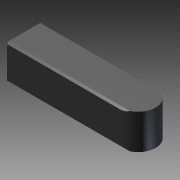
# Autodesk Inventor part: KEGS4-15
Saved by Autodesk Inventor 2011 SP1 (Build 150282100, 282)
## iProperties
Created: 2016-04-02
Part Number: KEGS4-15
Catalog Web Link: www.cadenas.de
Description: KED, KEDH, KEDS, KES, KESH, KESS, KEG, KEGH, KEGS-Parallel Keys
Vendor: MISUMI
Document SubType Name: Modeling
Designer: psAdmin
Manufacturer: MISUMI
Mass: 0.232054 g
Surface Area: 2.55242 cm^2
Volume: 0.232054 cm^3
Density: 1 g/cm^3
Category: PARTsolutions
Company: MISUMI
Title: KEGS4-15
Author: Cadenas PARTsolutions
Comments: Parallel Keys
PSOL_IDENT_0: {$CADENAS_DATA\23d-libs\misumi\metric\28_keys_magnets\kegh.prj},214 {VTYP=3D},{NB=KEGS4-15},{LINA=KE
PSOL_IDENT_1: GS4-15},{NN=KED, KEDH, KEDS, KES, KESH, KESS, KEG, KEGH, KEGS},{DATE=03.06.2015 11:36:45},{GEOMDATE=
PSOL_IDENT_2: 22.08.2013},{VERSION=},{LINEID=30},{LINESUBID=-1},{WBVAR=TYS,MAT,HARD,L,ALT1,LC}  {NB=KEGS4-15},{LIN
PSOL_IDENT_3: A=KEGS4-15},{KT=DUMMY},{PN=KEGS4-15},{PNALG=15},{TYS=KEG},{TYPEALG='KEDS','KEDS','KESS','KESS','KEGS'
PSOL_IDENT_4: ,'KEGS'},{MAT=S},{HARD=},{HARDALG='', '-'},{TS=600 or More},{B=4},{BTOL=0/-0.030},{L=15},{LALG=[8,10
PSOL_IDENT_5: ,12,15,16,18,20,25,30,35,40,45,50]},{LALG1=[8,10,12,15,16,20,25,30]},{ALT1=2},{LC=0},{LCALG=[0]},{LT
PSOL_IDENT_6: OL=0/-0.18},{H=4},{HTOL=0/-0.030},{C=0.16~0.25},{C1=0.200},{CALG=[0.16:0.25/0.01]}
NN: KED, KEDH, KEDS, KES, KESH, KESS, KEG, KEGH, KEGS
NT: Parallel Keys
NB: KEGS4-15
NBSYN: $PN.
LINA: KEGS4-15
PN: KEGS4-15
TYS: One Side Round
MAT: 316 Stainless Steel
HARD: -
TS: 600 or More
B: 4
BTOL: 0/-0.030
L: 15
ALT1: w/o LC (Changes Overall Length)
LC: 0
LTOL: 0/-0.18
H: 4
HTOL: 0/-0.030
C: 0.16~0.25
SUPPLIER: MISUMI
ARTICLENO: KEGS4-15
BOMINFO: KEGS4-15
CREATOR: CADENAS GmbH
Autodesk Inventor part; units mm, degrees
ref_plane "YZ Plane" through (0, 0, 0) normal (1, 0, 0) x (0, 1, 0)
ref_plane "XZ Plane" through (0, 0, 0) normal (0, 1, 0) x (-1, 0, 0)
ref_plane "XY Plane" through (0, 0, 0) normal (0, 0, 1) x (1, 0, 0)
sketch "Sketch_11" plane through (0, 0, 0) normal (0, 0, 1) x (1, 0, 0)
  line L0 (0, 0) -> (13, 0)
  arc A0 (13, 0) -> (15, 2) centre (13, 2) ccw
  arc A1 (15, 2) -> (13, 4) centre (13, 2) ccw
  line L1 (13, 4) -> (0, 4)
  line L2 (0, 4) -> (0, 0)
  constraints: 6 end point, 4 point on circle, 2 centre point
extrude "Extrusion1" add sketch "Sketch_11" along normal blind 4
sketch "Sketch_12" plane through (0, 0, 0) normal (1, 0, 0) x (0, 1, 0)
  line L0 (6, 6) -> (-2, 6)
  line L1 (-2, 6) -> (-2, -2)
  line L2 (-2, -2) -> (6, -2)
  line L3 (6, -2) -> (6, 6)
  line L4 (0.2, 4) -> (0, 3.8)
  line L5 (0, 3.8) -> (0, 0.2)
  line L6 (0, 0.2) -> (0.2, 0)
  line L7 (0.2, 0) -> (3.8, 0)
  line L8 (3.8, 0) -> (4, 0.2)
  line L9 (4, 0.2) -> (4, 3.8)
  line L10 (4, 3.8) -> (3.8, 4)
  line L11 (3.8, 4) -> (0.2, 4)
  constraints: 24 end point
extrude "Extrusion2" cut sketch "Sketch_12" along normal blind 15
body "Solid1"
